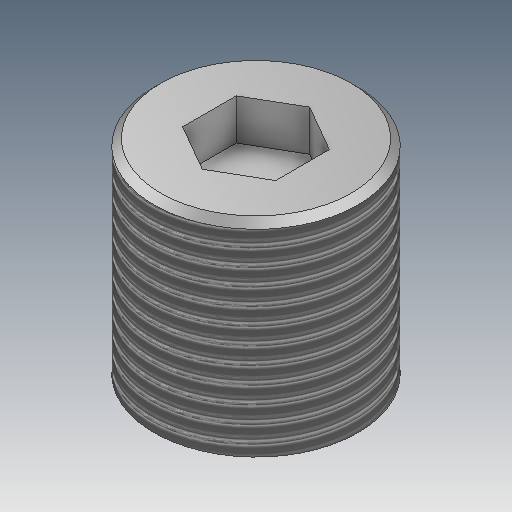
# Autodesk Inventor part: Tornillo Allen gusano M6 para Motor
Saved by Autodesk Inventor 2020.3 (Build 243373000, 373)
## iProperties
Created: 2020-05-17
Part Number: Tornillo Allen gusano M6 para Motor
Material: Genérico
Document SubType Name: Modeling
Designer: Pipi
Density: 1 g/cm^3
Appearance: Goma - Negro - Versión 1.1
Author: Pipi
Autodesk Inventor part; units mm, degrees
ref_plane "YZ Plane" through (0, 0, 0) normal (1, 0, 0) x (0, 1, 0)
ref_plane "XZ Plane" through (0, 0, 0) normal (0, 1, 0) x (-1, 0, 0)
ref_plane "XY Plane" through (0, 0, 0) normal (0, 0, 1) x (1, 0, 0)
sketch "Boceto1" plane through (0, 0, 0) normal (0, 1, 0) x (-1, 0, 0)
  circle A0 centre (10.9374, 23.9581) radius 3
  point P0 (0, 0)
  dimension "d0" = 6
  constraints: 1 centre point
  measures "d0" diameter of A0
extrude "Extrusión1" add sketch "Boceto1" along normal blind 6
sketch "Boceto2" plane through (-10.9374, 6, 23.9581) normal (0, 1, 0) x (1, 0, 0)
  line L0 (0, 1.58) -> (1.3683, 0.79)
  line L1 (1.3683, 0.79) -> (1.3683, -0.79)
  line L2 (1.3683, -0.79) -> (0, -1.58)
  line L3 (0, -1.58) -> (-1.3683, -0.79)
  line L4 (-1.3683, -0.79) -> (-1.3683, 0.79)
  line L5 (-1.3683, 0.79) -> (0, 1.58)
  circle A0 centre (0, 0) radius 3 projected
  line L6 (-3, 0) -> (0, 0)
  point P0 (10.9374, 23.9581)
  dimension "d11" = 1.58
  dimension "d12" = 1.58
  constraints: 14 end point, 1 horizontal, 1 horizontal alignment, 1 other
  measures "d11" distance of L2.end L3.end
  measures "d12" distance from line of L0.start L6
extrude "Extrusión2" cut sketch "Boceto2" against normal blind 1.2 contours L0 L1 L2 L3 L4 L5
thread "Thread2" size "M6x0.5" class "6g" standard "ISO Metric profile" length 7
chamfer "Chamfer1" distance 0.2 angle 45 1 edges at (-7.9374, 6, 23.9581)
